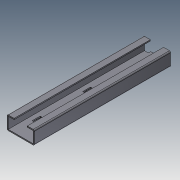
# Autodesk Inventor part: opstaand C-profiel van poot
Saved by Autodesk Inventor 2015 (Build 190159000, 159)
## iProperties
Created: 2007-07-03
Part Number: opstaand C-profiel van poot
Material: Steel, Mild
Document SubType Name: Sheet Metal
Designer: kurt
Manufacturer: Standard
Standards Organization: Custom
Density: 1 g/cm^3
Sheet Metal Rule: Default
Appearance: Steel
Author: kurt
Autodesk Inventor part; units mm, degrees
ref_plane "YZ Plane" through (0, 0, 0) normal (1, 0, 0) x (0, 1, 0)
ref_plane "XZ Plane" through (0, 0, 0) normal (0, 1, 0) x (-1, 0, 0)
ref_plane "XY Plane" through (0, 0, 0) normal (0, 0, 1) x (1, 0, 0)
sketch "Sketch1" plane through (0, 0, 0) normal (0, 0, 1) x (1, 0, 0)
  line L0 (-32, 0) -> (32, 0)
  line L1 (32, 0) -> (32, 350)
  line L2 (-32, 350) -> (-32, 0)
  line L3 (-22, 350) -> (-22, 356)
  line L4 (-22, 356) -> (22, 356)
  line L5 (22, 356) -> (22, 350)
  line L6 (32, 350) -> (22, 350)
  line L7 (-22, 350) -> (-32, 350)
  point P0 (0, 0)
  point P1 (0, 0)
  dimension "d42" = 350
  dimension "d46" = 10
  dimension "d47" = 10
  dimension "d48" = 64
  dimension "d49" = 6
  dimension "d50" = 64
  measures "d42" distance of L0.end L1.end
  measures "d46" horizontal distance of L4.end L1.end
  measures "d47" distance of L3.start L2.start
  measures "d48" distance of L1.end L2.start
  measures "d49" distance of L5.end L4.end
  measures "d50" distance of L0.start L0.end
extrude "Plate1" add sketch "Sketch1" along normal blind 3
sketch "Sketch2" plane through (-32, 0, 3) normal (1, 0, 0) x (0, 1, 0)
  line L0 (0, 0) -> (350, 0)
  line L1 (350, 0) -> (350, 29)
  line L2 (350, 29) -> (0, 29)
  line L3 (0, 29) -> (0, 0)
  constraints: 6 end point, 1 horizontal, 1 perpendicular, 1 vertical
sheet face with bend "Flange1" sketch "Sketch2" thickness 3 toward (-1, 0, 0) bend radius 0.001 relief straight relief width 3 relief depth 0.001
bend "Bend1"
sketch "Sketch3" plane through (32, 350, 3) normal (-1, 0, 0) x (0, -1, 0)
  line L0 (0, 0) -> (350, 0)
  line L1 (350, 0) -> (350, 29)
  line L2 (350, 29) -> (0, 29)
  line L3 (0, 29) -> (0, 0)
  constraints: 6 end point, 1 horizontal, 1 perpendicular, 1 vertical
sheet face with bend "Flange2" sketch "Sketch3" thickness 3 toward (1, 0, 0) bend radius 0.001 relief straight relief width 3 relief depth 0.001
bend "Bend2"
sketch "Sketch4" plane through (-32, 0, 32) normal (0, 0, -1) x (0, 1, 0)
  line L0 (0, 0) -> (350, 0)
  line L1 (350, 0) -> (350, 15)
  line L2 (350, 15) -> (0, 15)
  line L3 (0, 15) -> (0, 0)
  constraints: 6 end point, 1 horizontal, 1 perpendicular, 1 vertical
sheet face with bend "Flange3" sketch "Sketch4" thickness 3 toward (0, 0, 1) bend radius 0.001 relief straight relief width 3 relief depth 0.001
bend "Bend3"
sketch "Sketch5" plane through (32, 350, 32) normal (0, 0, -1) x (0, -1, 0)
  line L0 (0, 0) -> (350, 0)
  line L1 (350, 0) -> (350, 15)
  line L2 (350, 15) -> (0, 15)
  line L3 (0, 15) -> (0, 0)
  constraints: 6 end point, 1 horizontal, 1 perpendicular, 1 vertical
sheet face with bend "Flange4" sketch "Sketch5" thickness 3 toward (0, 0, 1) bend radius 0.001 relief straight relief width 3 relief depth 0.001
bend "Bend4"
sketch "Sketch6" plane through (-31.999, 0, 0) normal (0, 0, -1) x (-1, 0, 0)
  line L0 (-11.499, 200) -> (-15.499, 200)
  line L1 (-15.499, 200) -> (-15.499, 179.5)
  line L2 (-15.499, 179.5) -> (-11.499, 179.5)
  line L3 (-11.499, 179.5) -> (-11.499, 200)
  line L4 (-31.999, -35.6) -> (-31.999, 462.8) construction
  line L5 (-48.499, 179.5) -> (-52.499, 179.5)
  line L6 (-52.499, 179.5) -> (-52.499, 200)
  line L7 (-52.499, 200) -> (-48.499, 200)
  line L8 (-48.499, 200) -> (-48.499, 179.5)
  circle A0 centre (-31.999, 196) radius 4.5
  line L9 (-11.499, 70.5) -> (-15.499, 70.5)
  line L10 (-15.499, 70.5) -> (-15.499, 50)
  line L11 (-15.499, 50) -> (-11.499, 50)
  line L12 (-11.499, 50) -> (-11.499, 70.5)
  line L13 (-48.499, 70.5) -> (-52.499, 70.5)
  line L14 (-52.499, 70.5) -> (-52.499, 50)
  line L15 (-52.499, 50) -> (-48.499, 50)
  line L16 (-48.499, 50) -> (-48.499, 70.5)
  circle A1 centre (-31.999, 66.5) radius 4.5
  point P0 (0, 350)
  point P1 (0, 0)
  dimension "d33" = 4
  dimension "d34" = 20.5
  dimension "d35" = 4
  dimension "d36" = 20.5
  dimension "d37" = 0
  dimension "d38" = 33
  dimension "d45" = 150
  dimension "d51" = 4
  dimension "d52" = 9
  dimension "d62" = 20.5
  dimension "d63" = 4
  dimension "d64" = 9
  dimension "d65" = 20.5
  dimension "d66" = 4
  dimension "d68" = 4
  dimension "d69" = 0
  dimension "d71" = 50
  dimension "d72" = 33
  dimension "d73" = 16.5
  constraints: 32 end point, 8 parallel, 4 horizontal, 4 perpendicular, 2 centre point, 2 point on line, 1 other
  measures "d33" distance of L0.start L0.end
  measures "d34" distance of L2.end L0.start
  measures "d35" distance of L6.end L7.end
  measures "d36" distance of L5.end L6.end
  measures "d37" vertical distance of L0.end L7.end
  measures "d38" distance of L5.start L1.end
  measures "d45" vertical distance of point (0, 350) L0.start
  measures "d51" vertical distance of L0.end A0.centre
  measures "d52" diameter of A0
  measures "d62" distance of L11.end L9.start
  measures "d63" distance of L10.end L11.end
  measures "d64" diameter of A1
  measures "d65" distance of L13.end L14.end
  measures "d66" distance of L14.end L15.end
  measures "d68" vertical distance of L9.start A1.centre
  measures "d69" vertical distance of L13.start L9.start
  measures "d71" vertical distance of point (0, 0) L11.end
  measures "d72" distance of L9.end L13.start
  measures "d73" distance from line of L4 L9.end
extrude "Cut1" cut sketch "Sketch6" against normal blind 4
ref_plane "Work Plane4" through (35, 175, 31.999) normal (0, -1, 0) x (1, 0, 0)
ref_plane "Work Plane6" through (0, 0, 3) normal (1, 0, 0) x (0, 0, -1)
equation "\"d5\" = BendReliefWidth"
equation "\"d7\" = MinimumRemnant"
equation "\"d11\" = BendRadius"
equation "\"d6\" = BendReliefDepth"
equation "\"d8\" = BendRadius"
equation "\"d12\" = BendReliefWidth"
equation "\"d14\" = MinimumRemnant"
equation "\"d18\" = BendRadius"
equation "\"d13\" = BendReliefDepth"
equation "\"d15\" = BendRadius"
equation "\"d19\" = BendReliefWidth"
equation "\"d21\" = MinimumRemnant"
equation "\"d25\" = BendRadius"
equation "\"d20\" = BendReliefDepth"
equation "\"d22\" = BendRadius"
equation "\"d26\" = BendReliefWidth"
equation "\"d28\" = MinimumRemnant"
equation "\"d32\" = BendRadius"
equation "\"d27\" = BendReliefDepth"
equation "\"d29\" = BendRadius"
equation "\"BendReliefWidth\" = Thickness"
equation "\"CornerReliefSize\" = 4 * Thickness"
equation "\"MinimumRemnant\" = 2 * Thickness"
equation "\"TransitionRadius\" = BendRadius"
equation "\"d4\" = BendRadius"
equation "\"JacobiRadiusSize\" = Thickness"
equation "\"GapSize\" = Thickness"
equation "\"BendRadius\" = 0.001"
equation "\"BendReliefDepth\" = 0.001"
equation "\"Thickness\" = 3"
body "Solid1"
